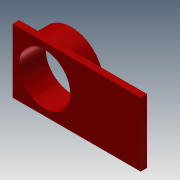
# Autodesk Inventor part: HbThumbMetacarpalPhalanxCover01
Saved by Autodesk Inventor 2015 SP1 (Build 190203100, 203)
## iProperties
Created: 2015-09-12
Part Number: HbThumbMetacarpalPhalanxCover01
Material: ABS プラスチック
Document SubType Name: Modeling
Designer: Yamaura
Density: 1.06 g/cm^3
Appearance: 滑らか - 赤
Author: Yamaura
Autodesk Inventor part; units mm, degrees
ref_plane "YZ Plane" through (0, 0, 0) normal (1, 0, 0) x (0, 1, 0)
ref_plane "XZ Plane" through (0, 0, 0) normal (0, 1, 0) x (-1, 0, 0)
ref_plane "XY Plane" through (0, 0, 0) normal (0, 0, 1) x (1, 0, 0)
sketch "スケッチ1" plane through (0, 0, 0) normal (0, 0, 1) x (1, 0, 0)
  circle A0 centre (0, 0) radius 8
  line L0 (-10, 10) -> (30, 10)
  line L1 (30, 10) -> (30, -10)
  line L2 (30, -10) -> (-10, -10)
  line L3 (-10, -10) -> (-10, 10)
  dimension "d0" = 16
  dimension "d1" = 10
  dimension "d2" = 10
  dimension "d3" = 20
  dimension "d4" = 30
  constraints: 8 end point, 2 parallel, 1 centre point, 1 coincident, 1 horizontal, 1 perpendicular
  measures "d0" diameter of A0
  measures "d1" distance from line of L3 point (0, 0)
  measures "d2" distance from line of L0 point (0, 0)
  measures "d3" distance of L2.end L0.start
  measures "d4" distance from line of L1 point (0, 0)
extrude "押し出し1" add sketch "スケッチ1" along normal blind 2
sketch "スケッチ2" plane through (0, 0, 0) normal (0, 0, 1) x (1, 0, 0)
  circle A0 centre (0, 0) radius 8
  circle A1 centre (0, 0) radius 10
  dimension "d7" = 16
  dimension "d8" = 20
  constraints: 2 centre point, 2 coincident
  measures "d7" diameter of A0
  measures "d8" diameter of A1
extrude "押し出し2" add sketch "スケッチ2" against normal blind 6.3
